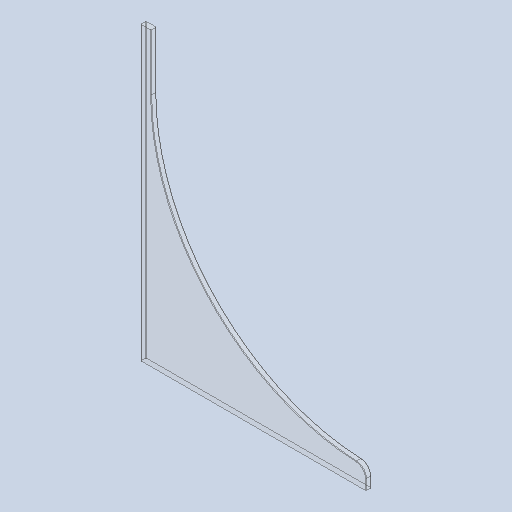
# Autodesk Inventor part: IndexCurveRail
Saved by Autodesk Inventor 2022 (Build 260153000, 153)
## iProperties
Created: 2022-01-14
Part Number: IndexCurveRail
Material: Polycarbonate, Clear
Document SubType Name: Modeling
Designer: tagaz
Density: 1.2 g/cm^3
Appearance: Polycarbonate - Clear
Author: tagaz
Autodesk Inventor part; units mm, degrees
ref_plane "YZ Plane" through (0, 0, 0) normal (1, 0, 0) x (0, 1, 0)
ref_plane "XZ Plane" through (0, 0, 0) normal (0, 1, 0) x (-1, 0, 0)
ref_plane "XY Plane" through (0, 0, 0) normal (0, 0, 1) x (1, 0, 0)
sketch "Sketch1" plane through (0, 0, 0) normal (0, 0, 1) x (1, 0, 0)
  arc A0 (-38.1, 0) -> (0, -38.1) centre (0, 0) ccw
  arc A1 (-266.6279, -6.2023) -> (-17.78, -266.1067) centre (0, 0) ccw
  line L0 (-272.9762, 0) -> (-273.05, 0)
  line L1 (0, -292.1) -> (-279.4, -292.1)
  line L2 (-279.4, -292.1) -> (-279.4, -6.35)
  arc A2 (-273.05, 0) -> (-279.4, -6.35) centre (-273.05, -6.35) ccw
  arc A3 (-266.6279, -6.2023) -> (-266.7, -5.3844) centre (-272.9762, -6.35) ccw
  arc A4 (-17.78, -266.1067) -> (-12.1227, -266.4243) centre (0, 0) ccw
  line L3 (0, -279.1112) -> (0, -292.1)
  arc A5 (0, -279.1112) -> (-12.1227, -266.4243) centre (-12.7, -279.1112) ccw
  line L4 (-273.05, 0) -> (-272.9762, 0)
  line L5 (-266.7, 0) -> (-266.7, 69.85)
  line L6 (-266.7, 69.85) -> (-279.4, 69.85)
  line L7 (-279.4, 69.85) -> (-279.4, 0)
  line L8 (-279.4, 0) -> (-279.4, -6.35)
  arc A6 (-266.7, 0) -> (-266.6279, -6.2023) centre (0, 0) ccw
  point P0 (0, -266.7)
  dimension "d0" = 76.2
  dimension "d21" = 228.6
  dimension "d24" = 292.1
  dimension "d25" = 279.4
  dimension "d27" = 6.35
  dimension "d34" = 266.7
  dimension "d35" = 12.7
  dimension "d36" = 12.9888
  dimension "d37" = 12.9888
  dimension "d39" = 266.7
  dimension "d40" = 12.7
  dimension "d41" = 266.7
  dimension "d42" = 69.85
  constraints: 18 end point, 15 point on circle, 8 tangent, 7 centre point, 4 point on line, 2 horizontal, 2 parallel, 2 perpendicular, 1 coincident, 1 equal radius, 1 vertical, 1 vertical alignment
  measures "d0" diameter of A0
  measures "d21" radial gap between concentric circles of A0 A1
  measures "d24" distance from line of point (0, 0) L1
  measures "d25" distance from line of point (0, 0) L2
  measures "d27" radius of A2
  measures "d34" radius of A4
  measures "d35" radius of A5
  measures "d36" distance from line of L1 A5.centre
  measures "d37" distance of L3.start L1.start
  measures "d39" distance of point (0, 0) A6.start
  measures "d40" distance of L5.end L6.end
  measures "d41" radius of A6
  measures "d42" distance from line of L0.end L6
extrude "Extrusion1" add sketch "Sketch1" along normal blind 6.35
fillet "Fillet3" radius 0.635 12 edges at (-279.4, -149.225, 6.35) (-279.4, -3.175, 6.35) (-279.4, 34.925, 6.35) (-266.682, -3.1014, 6.35) (-192.6383, -184.4434, 6.35) (-14.9522, -266.2805, 6.35) (-279.4, -149.225, 0) (-279.4, -3.175, 0) (-279.4, 34.925, 0) (-266.682, -3.1014, 0) (-192.6383, -184.4434, 0) (-14.9522, -266.2805, 0)
body "Solid1"
